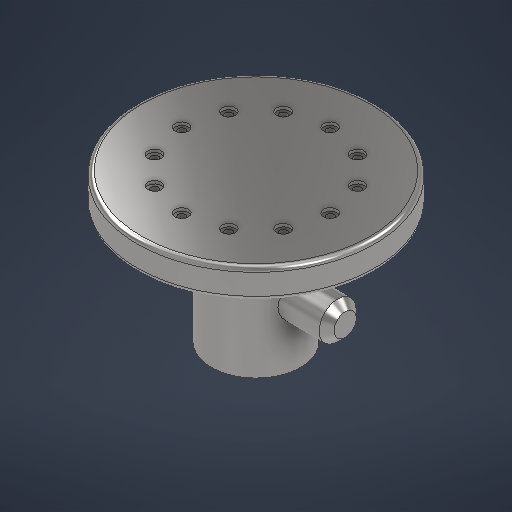
# Autodesk Inventor part: ensayo10
Saved by Autodesk Inventor 2026.2 (Build 302298000, 298)
## iProperties
Created: 2025-12-23
Part Number: ensayo10
Material: Acero inoxidable
Document SubType Name: Modeling
Designer: vicho
Mass: 5107.04 g
Surface Area: 674.644 cm^2
Volume: 638.38 cm^3
Density: 8 g/cm^3
Appearance: Semipulido
Author: vicho
Autodesk Inventor part; units mm, degrees
ref_plane "XY Plane" through (0, 0, 0) normal (0, 0, 1) x (1, 0, 0)
sketch "Boceto1" plane through (0, 0, 0) normal (0, 1, 0) x (-1, 0, 0)
  point P0 (0, 0)
sketch "Boceto2" plane through (0, 0, 0) normal (0, 1, 0) x (-1, 0, 0)
  line L0 (203.0537, 0) -> (-223.0639, 0) construction
  line L1 (0, 330.3943) -> (0, -330.3943) construction
  circle A0 centre (0, 0) radius 80
  circle A1 centre (0, 0) radius 50 construction
  point P0 (0, 50)
  dimension "d1" = 100
  dimension "d0" = 160
  constraints: 4 end point, 2 coincident, 2 horizontal, 2 vertical, 1 centre point, 1 point on line, 1 symmetric about line, 1 vertical alignment, 2 other
  measures "d0" diameter of A0
extrude "Extrusión1" add sketch "Boceto2" along normal blind 20
sketch "Boceto3" plane through (0, 20, 0) normal (0, 1, 0) x (1, 0, 0)
  circle A0 centre (0, 0) radius 50 construction
  point P0 (0, 50)
  point P1 (-25, 43.3013)
  point P2 (-43.3013, 25)
  point P3 (-50, 0)
  point P4 (-43.3013, -25)
  point P5 (-25, -43.3013)
  point P6 (0, -50)
  point P7 (25, -43.3013)
  point P8 (43.3013, -25)
  point P9 (50, 0)
  point P10 (43.3013, 25)
  point P11 (25, 43.3013)
  dimension "d4" = 100
  dimension "d14" = 360
  constraints: 1 coincident, 1 vertical alignment, 15 other
hole "Agujero1" at (0, 20, -50) direction (0, -1, 0) diameter 5 depth 6 tip angle 118 counterbore diameter 9 counterbore depth 2
hole "Agujero2" at (25, 20, -43.3013) at (43.3013, 20, -25) at (-25, 20, -43.3013) at (-43.3013, 20, -25) at (-50, 20, 0) at (-43.3013, 20, 25) at (-25, 20, 43.3013) at (0, 20, 50) at (25, 20, 43.3013) at (43.3013, 20, 25) at (50, 20, 0) direction (0, -1, 0) diameter 5 depth 6 tip angle 118 counterbore diameter 9 counterbore depth 2
fillet "Empalme1" radius 3 2 edges at (80, 20, 0) (80, 0, 0)
ref_plane "Plano de trabajo1" through (0, -80, 0) normal (0, 1, 0) x (-1, 0, 0)
sketch "Boceto4" plane through (0, -80, 0) normal (0, 1, 0) x (-1, 0, 0)
  circle A0 centre (0, 0) radius 30
  dimension "d25" = 60
  constraints: 1 centre point, 1 coincident
  measures "d25" diameter of A0
extrude "Extrusión2" add sketch "Boceto4" along normal up to next
fillet "Empalme2" radius 3 1 edges at (30, 0, 0)
ref_plane "Plano de trabajo2" through (60, 0, 0) normal (1, 0, 0) x (0, 1, 0)
sketch "Boceto5" plane through (60, 0, 0) normal (1, 0, 0) x (0, 1, 0)
  line L0 (76.488, 0) -> (-111.6725, 0) construction
  line L1 (0, 102.7061) -> (0, -141.7051) construction
  circle A0 centre (-40, 0) radius 12.5
  line L2 (-80, -30) -> (-80, 30) projected
  point P0 (0, 0)
  dimension "d30" = 25
  dimension "d31" = 40
  dimension "d32" = 80
  dimension "d33" = 0
  dimension "d34" = 156.488
  dimension "d35" = 31.6725
  dimension "d36" = 102.7061
  dimension "d37" = 141.7051
  constraints: 4 end point, 1 centre point, 1 horizontal, 1 point on line, 1 vertical
  measures "d30" diameter of A0
  measures "d31" distance from line of L2 A0.centre
  measures "d32" distance between parallel lines of L1 L2
  measures "d33" distance from line of point (0, 0) L0
  measures "d34" distance from line of L0.start L2
  measures "d35" distance from line of L0.end L2
  measures "d36" distance from line of L1.start L0
  measures "d37" distance from line of L1.end L0
extrude "Extrusión3" add sketch "Boceto5" against normal up to next
chamfer "Chaflán1" distance 5 angle 45 1 edges at (60, -52.5, 0)
shell "Vaciado1" thickness 6 removed faces 1 at (-9.4188, -80, 0)
